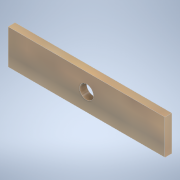
# Autodesk Inventor part: Moving eyebrow2
Saved by Autodesk Inventor 2021 (Build 250183000, 183)
## iProperties
Created: 2023-06-07
Part Number: Moving eyebrow2
Material: Wood (Maple)
Document SubType Name: Modeling
Designer: shrus
Density: 0.67 g/cm^3
Appearance: Natural Maple - Glossy Dark Tint
Author: shrus
Autodesk Inventor part; units mm, degrees
ref_plane "YZ Plane" through (0, 0, 0) normal (1, 0, 0) x (0, 1, 0)
ref_plane "XZ Plane" through (0, 0, 0) normal (0, 1, 0) x (-1, 0, 0)
ref_plane "XY Plane" through (0, 0, 0) normal (0, 0, 1) x (1, 0, 0)
sketch "Sketch1" plane through (0, 0, 0) normal (0, 0, 1) x (1, 0, 0)
  line L0 (-15.6214, 5.6366) -> (29.3786, 5.6366)
  line L1 (29.3786, 5.6366) -> (29.3786, -4.3634)
  line L2 (29.3786, -4.3634) -> (-15.6214, -4.3634)
  line L3 (-15.6214, -4.3634) -> (-15.6214, 5.6366)
  point P0 (0, 0)
  dimension "d1" = 45
  dimension "d2" = 10
  constraints: 8 end point, 3 perpendicular, 1 horizontal
  measures "d1" distance of L0.start L0.end
  measures "d2" distance of L0.end L1.end
extrude "Extrusion1" add sketch "Sketch1" along normal blind 2
sketch "Sketch2" plane through (0, 0, 2) normal (0, 0, 1) x (1, 0, 0)
  line L0 (-15.6214, 5.6366) -> (-15.6214, -4.3634) projected
  circle A0 centre (6.8786, 0.6366) radius 2
  point P0 (0, 0)
  dimension "d6" = 4
  constraints: 1 centre point
  measures "d6" diameter of A0
extrude "Extrusion2" cut sketch "Sketch2" against normal blind 2
body "Solid1"
